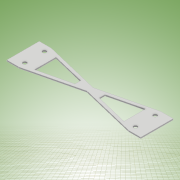
# Autodesk Inventor part: drill guide
Saved by Autodesk Inventor 2017 (Build 210142000, 142)
## iProperties
Created: 2018-06-07
Part Number: drill guide
Material: Generic
Document SubType Name: Modeling
Designer: Spark Electronics
Density: 1 g/cm^3
Appearance: Default
Author: Spark Electronics
Autodesk Inventor part; units mm, degrees
ref_plane "YZ Plane" through (0, 0, 0) normal (1, 0, 0) x (0, 1, 0)
ref_plane "XZ Plane" through (0, 0, 0) normal (0, 1, 0) x (-1, 0, 0)
ref_plane "XY Plane" through (0, 0, 0) normal (0, 0, 1) x (1, 0, 0)
sketch "Sketch1" plane through (0, 0, 0) normal (0, 0, 1) x (1, 0, 0)
  line L0 (-52.5, -12.7) -> (-52.5, 12.7)
  line L1 (43, 12.7) -> (52.5, 12.7)
  line L2 (52.5, 12.7) -> (52.5, -12.7)
  line L3 (52.5, -12.7) -> (-52.5, 12.7) construction
  line L4 (-52.5, -12.7) -> (-43, -12.7)
  line L5 (-43, 12.7) -> (-52.5, 12.7)
  line L6 (-52.5, 12.7) -> (-52.5, -12.7)
  line L7 (52.5, -12.7) -> (43.7955, -12.7)
  line L8 (43.7955, 12.7) -> (52.5, 12.7)
  line L9 (52.5, 12.7) -> (52.5, -12.7)
  circle A0 centre (-43.423, 7.694) radius 1.5
  circle A1 centre (-43.423, -7.706) radius 1.5
  line L10 (0, 19) -> (0, -21) construction
  line L11 (52.5, -12.7) -> (52.5, 12.7)
  line L12 (52.5, -12.7) -> (43, -12.7)
  line L13 (43, 12.7) -> (52.5, 12.7)
  line L14 (52.5, 12.7) -> (52.5, -12.7)
  circle A2 centre (43.423, 7.694) radius 1.5
  circle A3 centre (43.423, -7.706) radius 1.5
  line L15 (-43, 12.7) -> (0, 2.2981)
  line L16 (0, 2.2981) -> (0, 0)
  line L17 (-52.5, 0) -> (75, 0) construction
  line L18 (-43, -12.7) -> (0, -2.2981)
  line L19 (0, -2.2981) -> (0, 0)
  line L20 (43, 12.7) -> (0, 2.2981)
  line L21 (43, -12.7) -> (0, -2.2981)
  line L22 (-35.158, 8.5049) -> (-35.158, 0)
  line L23 (-35.158, 8.5049) -> (-9.4754, 2.2921)
  line L24 (-9.4754, 0) -> (-9.4754, 2.2921)
  line L25 (52.5, 12.7) -> (-52.5, -12.7) construction
  line L26 (-35.158, -8.5049) -> (-35.158, 0)
  line L27 (-9.4754, 0) -> (-9.4754, -2.2921)
  line L28 (-35.158, -8.5049) -> (-9.4754, -2.2921)
  line L29 (35.158, 8.5049) -> (35.158, 0)
  line L30 (35.158, 8.5049) -> (9.4754, 2.2921)
  line L31 (9.4754, 0) -> (9.4754, 2.2921)
  line L32 (35.158, -8.5049) -> (35.158, 0)
  line L33 (9.4754, 0) -> (9.4754, -2.2921)
  line L34 (35.158, -8.5049) -> (9.4754, -2.2921)
  line L35 (-43.423, 7.694) -> (43.423, 7.694) construction
  line L36 (-52.5, 12.7) -> (-43, 12.7)
  line L37 (0, 2.2981) -> (-43, 12.7)
  line L38 (0, 2.2981) -> (43, 12.7)
  line L39 (43, 12.7) -> (52.5, 12.7)
  line L40 (52.5, 12.7) -> (52.5, -12.7)
  line L41 (52.5, -12.7) -> (43, -12.7)
  line L42 (43, -12.7) -> (0, -2.2981)
  line L43 (0, -2.2981) -> (-43, -12.7)
  line L44 (-43, -12.7) -> (-52.5, -12.7)
  line L45 (-52.5, -12.7) -> (-52.5, 12.7)
  dimension "d0" = 105
  dimension "d1" = 15.4
  dimension "d4" = 9.077
  dimension "d5" = 3
  dimension "d6" = 3
  constraints: 92 end point, 17 symmetric about line, 11 point on line, 7 collinear, 6 parallel, 5 perpendicular, 4 centre point, 3 horizontal, 2 midpoint, 1 vertical, 2 other
  measures "d0" distance of L0.end L1.end
  measures "d1" distance of L35.start A1.centre
  measures "d4" distance from line of L0 L35.start
  measures "d5" diameter of A1
  measures "d6" diameter of A0
extrude "Extrusion1" add sketch "Sketch1" along normal blind 1
body "Solid1"
